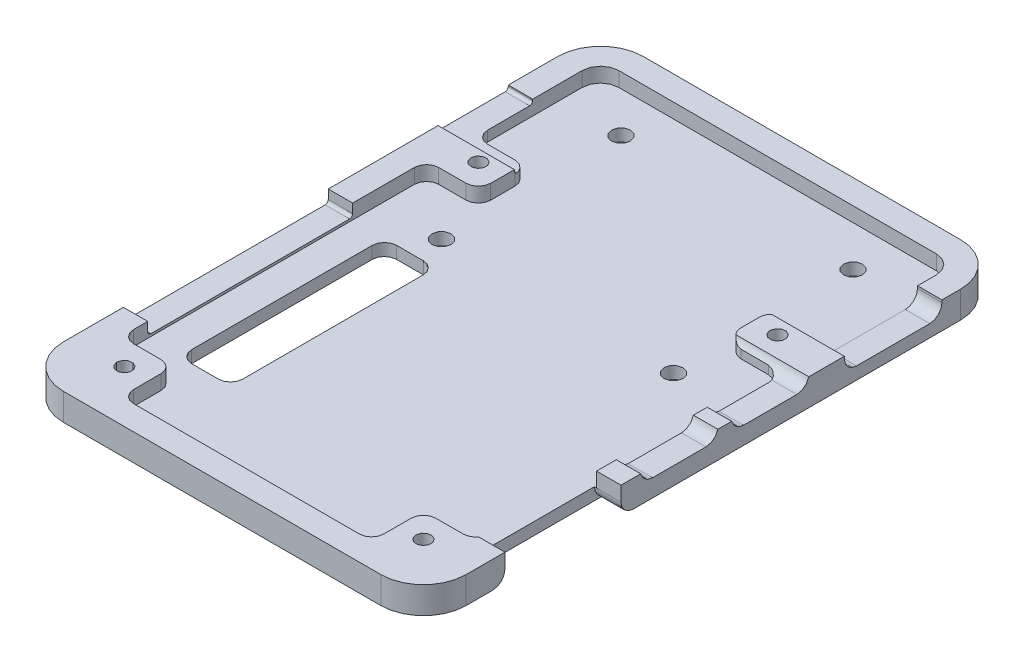
# Autodesk Inventor part: bottom
Saved by Autodesk Inventor 2021 (Build 250183000, 183)
## iProperties
Created: 2021-01-15
Part Number: bottom
Material: ABS Plastic
Document SubType Name: Modeling
Designer: User
Density: 1.06 g/cm^3
Appearance: Smooth - Black
Author: User
Autodesk Inventor part; units mm, degrees
ref_plane "YZ Plane" through (0, 0, 0) normal (1, 0, 0) x (0, 1, 0)
ref_plane "XZ Plane" through (0, 0, 0) normal (0, 1, 0) x (-1, 0, 0)
ref_plane "XY Plane" through (0, 0, 0) normal (0, 0, 1) x (1, 0, 0)
sketch "base_sketch" plane through (0, 0, 0) normal (0, 1, 0) x (-1, 0, 0)
  line L0 (-33, 47.5) -> (33, 47.5)
  line L1 (33, 47.5) -> (33, -47.5)
  line L2 (33, -47.5) -> (-33, -47.5)
  line L3 (-33, -47.5) -> (-33, 47.5)
  line L4 (-33, 47.5) -> (33, -47.5) construction
  line L5 (33, 47.5) -> (-33, -47.5) construction
  circle A0 centre (24.5, 39) radius 1.25
  circle A1 centre (24.5, -19) radius 1.25
  circle A2 centre (-24.5, 39) radius 1.25
  circle A3 centre (-24.5, -19) radius 1.25
  line L6 (29, 43.5) -> (-29, 43.5)
  line L7 (-29, 43.5) -> (-29, -43.5)
  line L8 (-29, -43.5) -> (29, -43.5)
  line L9 (29, -43.5) -> (29, 43.5)
  line L10 (29, 43.5) -> (-29, -43.5) construction
  line L11 (-29, 43.5) -> (29, -43.5) construction
  line L12 (-29, 43.5) -> (-20.5, 43.5)
  line L13 (-20.5, 43.5) -> (-20.5, 35)
  line L14 (-20.5, 35) -> (-29, 35)
  line L15 (-29, 35) -> (-29, 43.5)
  line L16 (-29, -15) -> (-20.5, -15)
  line L17 (-20.5, -15) -> (-20.5, -22)
  line L18 (-20.5, -22) -> (-29, -22)
  line L19 (-29, -22) -> (-29, -15)
  line L20 (29, -15) -> (20.5, -15)
  line L21 (20.5, -15) -> (20.5, -23)
  line L22 (20.5, -23) -> (29, -23)
  line L23 (29, -23) -> (29, -15)
  line L24 (29, 43.5) -> (20.5, 43.5)
  line L25 (20.5, 43.5) -> (20.5, 35)
  line L26 (20.5, 35) -> (29, 35)
  line L27 (29, 35) -> (29, 43.5)
  point P0 (0, 0)
  point P1 (-29, -22)
  dimension "d0" = 66
  dimension "d1" = 95
  dimension "d14" = 2.5
  dimension "d17" = 58
  dimension "d20" = 49
  dimension "d24" = 24.5
  dimension "d25" = 58
  dimension "d26" = 87
  dimension "d27" = 4.5
  dimension "d42" = 4
  dimension "d43" = 4
  dimension "d44" = 4
  dimension "d45" = 4
  dimension "d46" = 4
  dimension "d47" = 4
  dimension "d48" = 4
  dimension "d49" = 4
  dimension "d50" = 3
  constraints: 56 end point, 12 parallel, 7 horizontal, 6 perpendicular, 4 centre point, 4 midpoint, 3 point on line, 1 vertical, 6 other
  measures "d0" distance of L1.end L2.end
  measures "d1" distance of L0.end L1.end
  measures "d14" diameter of A0
  measures "d17" distance of A0.centre A1.centre
  measures "d20" distance of A0.centre A2.centre
  measures "d24" horizontal distance of point (0, 0) A0.centre
  measures "d25" distance of L8.end L7.end
  measures "d26" distance of L7.end L6.end
  measures "d27" distance from line of L6 A0.centre
  measures "d42" distance from line of L21 A1.centre
  measures "d43" distance from line of A1.centre L20
  measures "d44" distance from line of A1.centre L22
  measures "d45" distance from line of L25 A0.centre
  measures "d46" distance from line of A0.centre L26
  measures "d47" distance from line of A2.centre L14
  measures "d48" distance from line of A2.centre L13
  measures "d49" distance from line of L17 A3.centre
  measures "d50" distance from line of A3.centre L18
extrude "base" add sketch "base_sketch" along normal blind 2 contours L25 L26 L9 L20 L21 L22 L8 L7 L18 L17 L16 L14 L13 L6
extrude "walls" add sketch "base_sketch" along normal blind 4.4 contours L0 L1 L2 L3
extrude "standoffs" add sketch "base_sketch" along normal blind 4.4 contours L9 L26 L25 L6 | L13 L14 L7 L6 | L9 L22 L21 L20 | L16 L17 L18 L7
fillet "inside" radius 3 2 edges at (-29, 3.2, -43.5) (29, 3.2, -43.5)
fillet "outside" radius 7 4 edges at (-33, 2.2, -47.5) (33, 2.2, -47.5) (33, 2.2, 47.5) (-33, 2.2, 47.5)
fillet "fillet_standoffs" radius 2 14 edges at (-29, 3.2, -15) (-20.5, 3.2, -15) (-20.5, 3.2, -23) (-29, 3.2, -23) (-29, 3.2, 35) (-20.5, 3.2, 35) (-20.5, 3.2, 43.5) (20.5, 3.2, 35) (20.5, 3.2, -22) (20.5, 3.2, -15) (29, 3.2, -22) (29, 3.2, 35) (20.5, 3.2, 43.5) (29, 3.2, -15)
sketch "cutout_usbc_data_sketch" plane through (33, 0, 40.5) normal (1, 0, 0) x (0, 0, -1)
  line L0 (7.5, 4.4) -> (53.5, 4.4) projected
  line L1 (28.53, 4.4) -> (41.27, 4.4)
  line L2 (41.27, 4.4) -> (41.27, 4.87)
  line L3 (39.27, 2.87) -> (30.53, 2.87)
  line L4 (28.53, 4.87) -> (28.53, 4.4)
  line L5 (88, 0) -> (88, 4.4) projected
  arc A0 (28.53, 4.87) -> (30.53, 2.87) centre (30.53, 4.87) ccw
  arc A1 (39.27, 2.87) -> (41.27, 4.87) centre (39.27, 4.87) ccw
  point P0 (40.5, 0)
  point P1 (41.27, 2.87)
  point P2 (28.53, 2.87)
  point P3 (41.214, 4.4)
  point P4 (28.586, 4.4)
  dimension "d60" = 1.53
  dimension "d61" = 46.73
  dimension "d62" = 12.74
  dimension "d63" = 2
  constraints: 8 end point, 5 point on line, 4 point on circle, 4 tangent, 2 centre point, 2 parallel, 1 equal radius, 1 horizontal, 1 perpendicular
  measures "d60" distance of L1.end point (41.27, 2.87)
  measures "d61" distance between parallel lines of L5 L2
  measures "d62" distance of point (41.27, 2.87) point (28.53, 2.87)
  measures "d63" radius of A0
extrude "cutout_usbc_data" cut sketch "cutout_usbc_data_sketch" against normal up to surface (4 mm away) contours L0 A1 L3 A0
sketch "cutout_usbc_pwr_sketch" plane through (33, 0, 40.5) normal (1, 0, 0) x (0, 0, -1)
  line L0 (7.5, 4.4) -> (53.5, 4.4) projected
  line L1 (43.43, 4.4) -> (56.17, 4.4)
  line L2 (56.17, 4.4) -> (56.17, 4.8682)
  line L3 (54.17, 2.8682) -> (45.43, 2.8682)
  line L4 (43.43, 4.8682) -> (43.43, 4.4)
  line L5 (88, 0) -> (88, 4.4) projected
  arc A0 (43.43, 4.8682) -> (45.43, 2.8682) centre (45.43, 4.8682) ccw
  arc A1 (54.17, 2.8682) -> (56.17, 4.8682) centre (54.17, 4.8682) ccw
  point P0 (40.5, 0)
  point P1 (56.17, 2.8682)
  point P2 (43.43, 2.8682)
  point P3 (56.1144, 4.4)
  point P4 (43.4856, 4.4)
  dimension "d66" = 31.83
  dimension "d67" = 12.74
  dimension "d68" = 1.5318
  dimension "d69" = 2
  constraints: 8 end point, 5 point on line, 4 point on circle, 4 tangent, 2 centre point, 2 parallel, 1 equal radius, 1 horizontal, 1 perpendicular
  measures "d66" distance between parallel lines of L5 L2
  measures "d67" distance of point (56.17, 2.868) point (43.43, 2.868)
  measures "d68" distance of point (43.43, 2.868) L1.start
  measures "d69" radius of A0
extrude "cutout_usbc_pwr" cut sketch "cutout_usbc_pwr_sketch" against normal up to surface (12.5 mm away) contours L0 L1 A1 L3 A0
sketch "cutout_hdmi_sketch" plane through (33, 0, 40.5) normal (1, 0, 0) x (0, 0, -1)
  line L0 (7.5, 4.4) -> (53.5, 4.4) projected
  line L1 (25.35, 4.4) -> (6.35, 4.4)
  line L2 (6.35, 4.4) -> (6.35, 0)
  line L3 (6.35, 0) -> (25.35, 0)
  line L4 (25.35, 0) -> (25.35, 4.4)
  line L5 (-7, 4.4) -> (-7, 0) projected
  point P0 (40.5, 0)
  point P1 (43.4856, 4.4)
  point P2 (7.5, 4.4)
  dimension "d72" = 19
  dimension "d73" = 13.35
  constraints: 8 end point, 2 parallel, 1 horizontal, 1 horizontal alignment, 1 perpendicular, 1 point on line
  measures "d72" distance of L2.end L3.end
  measures "d73" distance between parallel lines of L5 L2
extrude "cutout_hdmi" cut sketch "cutout_hdmi_sketch" against normal blind 4.364
fillet "cutout_hdmi_fillet" radius 2 2 edges at (30.818, 0, 34.15) (30.818, 0, 15.15)
sketch "cutout_microsd_sketch" plane through (33, 0, -40.5) normal (1, 0, 0) x (0, 0, -1)
  line L0 (-24.8856, 4.4) -> (0, 4.4) projected
  line L1 (-19.063, 4.4) -> (-3.068, 4.4)
  line L2 (-3.068, 4.4) -> (-3.068, 4.03)
  line L3 (-5.068, 2.03) -> (-17.063, 2.03)
  line L4 (-19.063, 4.03) -> (-19.063, 4.4)
  line L5 (7, 0) -> (7, 4.4) projected
  arc A0 (-19.063, 4.03) -> (-17.063, 2.03) centre (-17.063, 4.03) ccw
  arc A1 (-5.068, 2.03) -> (-3.068, 4.03) centre (-5.068, 4.03) ccw
  point P0 (-40.5, 0)
  point P1 (-3.068, 2.03)
  point P2 (-19.063, 2.03)
  point P3 (-3.068, 4.4)
  dimension "d78" = 10.068
  dimension "d79" = 15.995
  dimension "d80" = 2.37
  dimension "d81" = 2
  constraints: 8 end point, 5 point on line, 4 point on circle, 4 tangent, 2 centre point, 2 parallel, 1 equal radius, 1 horizontal, 1 perpendicular
  measures "d78" distance between parallel lines of L5 L2
  measures "d79" distance of point (-3.068, 2.03) point (-19.063, 2.03)
  measures "d80" distance of point (-19.063, 2.03) L1.start
  measures "d81" radius of A0
extrude "cutout_microsd" cut sketch "cutout_microsd_sketch" against normal blind 16.77
sketch "cutout_flatflex_sketch" plane through (-33, 0, -40.5) normal (-1, 0, 0) x (0, 0, 1)
  line L0 (73.5, 4.4) -> (27.5, 4.4) projected
  line L1 (37.599, 4.4) -> (71.172, 4.4)
  line L2 (71.172, 4.4) -> (71.172, 2.9)
  line L3 (70.672, 2.4) -> (38.099, 2.4)
  line L4 (37.599, 2.9) -> (37.599, 4.4)
  line L5 (88, 0) -> (88, 4.4) projected
  arc A0 (37.599, 2.9) -> (38.099, 2.4) centre (38.099, 2.9) ccw
  arc A1 (70.672, 2.4) -> (71.172, 2.9) centre (70.672, 2.9) ccw
  point P0 (40.5, 0)
  point P1 (71.172, 2.4)
  point P2 (37.599, 2.4)
  dimension "d85" = 16.828
  dimension "d86" = 33.573
  dimension "d87" = 2
  dimension "d90" = 0.5
  constraints: 8 end point, 5 point on line, 4 point on circle, 4 tangent, 2 centre point, 2 parallel, 1 equal radius, 1 horizontal, 1 perpendicular
  measures "d85" distance between parallel lines of L5 L2
  measures "d86" distance of point (71.172, 2.4) point (37.599, 2.4)
  measures "d87" distance of point (37.599, 2.4) L1.start
  measures "d90" radius of A0
extrude "cutout_flatflex" cut sketch "cutout_flatflex_sketch" against normal up to surface (12.5 mm away)
sketch "cutout_flatflex_below_sketch" plane through (0, 0, 0) normal (0, -1, 0) x (1, 0, 0)
  line L0 (-17.432, -2.901) -> (-21.8, -2.901)
  line L1 (-23.8, -0.901) -> (-23.8, 28.672)
  line L2 (-21.8, 30.672) -> (-17.432, 30.672)
  line L3 (-15.432, 28.672) -> (-15.432, -0.901)
  line L4 (-26, 47.5) -> (26, 47.5) projected
  line L5 (-33, -40.5) -> (-33, 40.5) projected
  arc A0 (-17.432, -2.901) -> (-15.432, -0.901) centre (-17.432, -0.901) ccw
  arc A1 (-23.8, -0.901) -> (-21.8, -2.901) centre (-21.8, -0.901) ccw
  arc A2 (-21.8, 30.672) -> (-23.8, 28.672) centre (-21.8, 28.672) ccw
  arc A3 (-15.432, 28.672) -> (-17.432, 30.672) centre (-17.432, 28.672) ccw
  point P0 (0, 0)
  point P1 (-15.432, -2.901)
  point P2 (-15.432, 30.672)
  dimension "d91" = 16.828
  dimension "d92" = 33.573
  dimension "d93" = 17.568
  dimension "d94" = 9.2
  dimension "d95" = 2
  constraints: 8 end point, 8 point on circle, 8 tangent, 4 centre point, 4 point on line, 3 equal radius, 2 parallel, 1 horizontal, 1 perpendicular
  measures "d91" distance between parallel lines of L4 L2
  measures "d92" distance of point (-15.432, 30.672) point (-15.432, -2.901)
  measures "d93" distance between parallel lines of L5 L3
  measures "d94" distance between parallel lines of L5 L1
  measures "d95" radius of A0
extrude "cutout_flatflex_below" cut sketch "cutout_flatflex_below_sketch" against normal up to surface (2 mm away)
sketch "cutout_microusb_sketch" plane through (-33, 0, -40.5) normal (-1, 0, 0) x (0, 0, 1)
  line L0 (0, 4.4) -> (37.599, 4.4) projected
  line L1 (8.107, 4.4) -> (19.606, 4.4)
  line L2 (19.606, 4.4) -> (19.606, 4.2)
  line L3 (19.106, 3.7) -> (8.607, 3.7)
  line L4 (8.107, 4.2) -> (8.107, 4.4)
  line L5 (88, 0) -> (88, 4.4) projected
  arc A0 (8.107, 4.2) -> (8.607, 3.7) centre (8.607, 4.2) ccw
  arc A1 (19.106, 3.7) -> (19.606, 4.2) centre (19.106, 4.2) ccw
  point P0 (40.5, 0)
  point P1 (19.606, 3.7)
  point P2 (8.107, 3.7)
  point P3 (19.5599, 4.4)
  point P4 (8.1531, 4.4)
  dimension "d98" = 68.394
  dimension "d99" = 11.499
  dimension "d100" = 0.7
  dimension "d101" = 0.5
  constraints: 8 end point, 5 point on line, 4 point on circle, 4 tangent, 2 centre point, 2 parallel, 1 equal radius, 1 horizontal, 1 perpendicular
  measures "d98" distance between parallel lines of L5 L2
  measures "d99" distance of point (19.606, 3.7) point (8.107, 3.7)
  measures "d100" distance of point (8.107, 3.7) L1.start
  measures "d101" radius of A0
extrude "cutout_microusb" cut sketch "cutout_microusb_sketch" against normal up to surface (12.5 mm away)
sketch "holes_mounting_sketch" plane through (0, 2, 0) normal (0, 1, 0) x (1, 0, 0)
  circle A0 centre (-19, 7.451) radius 1.55
  circle A1 centre (19, 7.451) radius 1.55
  line L0 (0, 0) -> (0, 26.6981) construction
  circle A2 centre (-19, 7.451) radius 3.55 construction
  line L1 (-21.8, 2.901) -> (-17.432, 2.901) construction
  circle A3 centre (-19, 36.851) radius 1.55
  circle A4 centre (19, 36.851) radius 1.55
  dimension "d104" = 3.1
  dimension "d105" = 2
  dimension "d106" = 38
  dimension "d107" = 4.55
  dimension "d108" = 3.1
  dimension "d111" = 29.4
  dimension "d112" = 3.1
  dimension "d113" = 3.1
  constraints: 5 centre point, 2 end point, 2 horizontal alignment, 2 vertical alignment, 1 coincident, 1 symmetric about line, 1 vertical
  measures "d104" diameter of A0
  measures "d105" radial gap between concentric circles of A0 A2
  measures "d106" diameter of A0.centre L0
  measures "d107" distance from line of A0.centre L1
  measures "d108" diameter of A1
  measures "d111" distance of A0.centre A3.centre
  measures "d112" diameter of A3
  measures "d113" diameter of A4
extrude "holes_mounting" cut sketch "holes_mounting_sketch" against normal up to surface (2 mm away)
equation "\"d14\" = hole"
equation "\"d24\" = 0.5 * d20"
equation "\"d44\" = d43"
equation "\"d108\" = d104"
equation "\"d112\" = d104"
equation "\"d113\" = d108"
equation "\"hole\" = 2.5"
body "Solid2"
